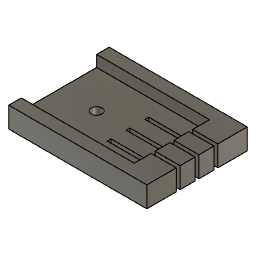
BristleCutGuide (Autodesk Fusion 360 design; units mm, degrees)
Autodesk Fusion 360 part; units mm, degrees
sketch "Main Body" plane through (0, 0, 0) normal (0, 0, 1) x (1, 0, 0)
  line L0 (9, 8) -> (-9, 8)
  line L1 (-9, 8) -> (-9, -8)
  line L2 (-9, -8) -> (9, -8)
  line L3 (9, -8) -> (9, 8)
  line L4 (9, 8) -> (-9, -8) construction
  line L5 (-9, 8) -> (9, -8) construction
  line L6 (9, 8) -> (13, 8)
  line L7 (13, 8) -> (13, -8)
  line L8 (13, -8) -> (9, -8)
  line L9 (9, -8) -> (9, 8)
  line L10 (9, 6) -> (-9, 6)
  line L11 (-9, -6) -> (9, -6)
  line L12 (2, 3.3) -> (13, 3.3)
  line L13 (13, 3.3) -> (13, 2.7)
  line L14 (13, 2.7) -> (2, 2.7)
  line L15 (2, 2.7) -> (2, 3.3)
  circle A0 centre (-3, 0) radius 0.85
  point P0 (2, 3)
  dimension "d4" = 18
  dimension "d5" = 4
  dimension "d7" = 16
  dimension "d8" = -2
  dimension "d9" = -2
  dimension "d10" = 0.6
  dimension "d11" = 7
  dimension "d12" = 3
  dimension "d26" = 1.7
  dimension "d27" = 6
  constraint horizontal L0
  constraint perpendicular L0 L1
  constraint parallel L0 L2
  constraint parallel L1 L3
  constraint coincident L4 origin
  constraint coincident L5 origin
  constraint horizontal L6
  constraint vertical L7
  constraint horizontal L8
  constraint vertical L9
  constraint coincident L2.end L3.start
  constraint horizontal L12
  constraint vertical L13
  constraint horizontal L14
  constraint vertical L15
  constraint coincident L7 L13.end
  constraint midpoint L15 P0
  constraint horizontal origin A0.centre
  measures "d4" distance of L0.start L0.end
  measures "d5" distance of L0.start L6.end
  measures "d7" distance of L0.end L1.end
  measures "d10" distance of L12 L14
  measures "d11" distance of L9 L12.start
  measures "d12" distance of L10 P0
  measures "d26" diameter of A0
  measures "d27" distance of L1 A0.centre
extrude "Base" add sketch "Main Body" against normal blind 1.5 contours L0 L1 L3 L9 L10 | L3 L6 L7 L9 L12 | L1 L3 L9 L10 L11 L12 L14 L15 | L3 L7 L9 L12 L13 L14 | L3 L9 L12 L14 L15 | L1 L2 L3 L9 L11 | L3 L7 L8 L9 L14 | A0
extrude "Guide" add sketch "Main Body" along normal blind 1.8 contours L0 L1 L3 L9 L10 | L3 L6 L7 L9 L12 | L3 L7 L9 L12 L13 L14 | L1 L2 L3 L9 L11 | L3 L7 L8 L9 L14
extrude "Bristle Cut" cut sketch "Main Body" along normal through all and the other way through all contours L3 L7 L9 L12 L13 L14 | L3 L9 L12 L14 L15
pattern_linear "Bristle Pattern" count 3 spacing 3 along (0, -1, 0) of "Bristle Cut"
extrude "Fixing Hole" cut sketch "Main Body" against normal through all contours A0
equation "SegmentLength = 18 mm" comment "Band Cut Length default 18mm"
equation "NumBristles = 4" comment "Number of Bristles per Segment"
equation "d4 = SegmentLength"
equation "BandWidth = 12 mm" comment "Width of Silicont Band"
equation "d7 = BandWidth + 4 mm"
equation "d11 = SegmentLength - 11 mm"
equation "d12 = BandWidth / NumBristles"
equation "d15 = BandThickness - 0.2 mm"
equation "d19 = NumBristles - 1"
equation "d21 = -BandWidth / NumBristles"
equation "BandThickness = 2 mm" comment "Thickness of band"
named bodies: "Bristle Cutting Guide"
